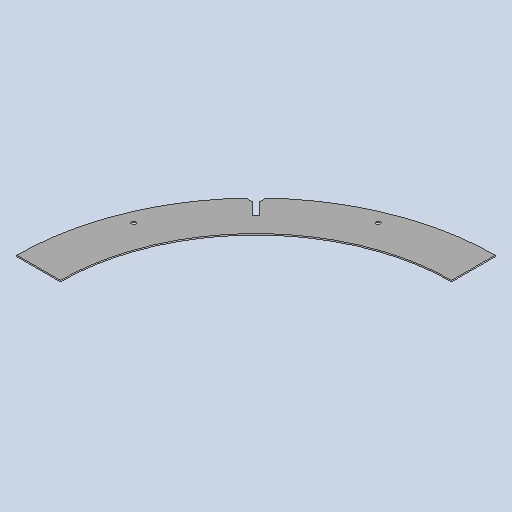
# Autodesk Inventor part: BSH 502 segment
Saved by Autodesk Inventor 2025 (Build 290162010, 162A)
## iProperties
Created: 2024-09-03
Part Number: BSH 502 segment
Material: Stainless Steel
Document SubType Name: Sheet Metal
Designer: pokla
Density: 8 g/cm^3
Flat Pattern Width: 55 cm
Flat Pattern Length: 55 cm
Flat Pattern Area: 3025 cm^2
Sheet Metal Rule: AISI304 3mm Die 32
Sheet Metal Width: 550.000 mm
Sheet Metal Length: 550.000 mm
Sheet Metal Area: 302500.000 mm^2
Appearance: Default
Mass: 1864.38 g
Surface Area: 1611.3 cm^2
Volume: 233.048 cm^3
Author: pokla
Autodesk Inventor part; units mm, degrees
ref_plane "YZ Plane" through (0, 0, 0) normal (1, 0, 0) x (0, 1, 0)
ref_plane "XZ Plane" through (0, 0, 0) normal (0, 1, 0) x (-1, 0, 0)
ref_plane "XY Plane" through (0, 0, 0) normal (0, 0, 1) x (1, 0, 0)
sketch "Sketch1" plane through (0, 0, 0) normal (0, 0, 1) x (1, 0, 0)
  arc A0 (0, 550) -> (-550, 0) centre (0, 0) ccw
  arc A1 (0, 450) -> (-450, 0) centre (0, 0) ccw
  line L0 (0, 550) -> (0, 450)
  line L1 (-450, 0) -> (-550, 0)
  point P0 (-500, 0)
  point P1 (0, 500)
  dimension "d0" = 1100
  dimension "d1" = 900
  measures "d0" diameter of A0
  measures "d1" diameter of A1
extrude "Plate1" add sketch "Sketch1" against normal blind 3
sketch "Sketch2" plane through (0, 0, 0) normal (0, 0, 1) x (1, 0, 0)
  line L0 (-550, 0) -> (-450, 0) projected
  arc A0 (0, 550) -> (-550, 0) centre (0, 0) ccw construction
  circle A1 centre (-480.4174, 198.9954) radius 5
  arc A2 (0, 450) -> (-450, 0) centre (0, 0) ccw construction
  circle A3 centre (0, 0) radius 520 construction
  line L1 (-480.4174, 198.9954) -> (0, 0) construction
  dimension "d17" = 1040
  dimension "d4" = 10
  dimension "d16" = 22.5
  constraints: 2 coincident, 2 end point, 1 centre point, 3 other
  measures "d4" diameter of A1
  measures "d16" angle of L1 L0
extrude "Cut1" cut sketch "Sketch2" against normal through all
pattern_circular "Circular Pattern1" count 2 over 45 about axis through (0, 0, 0) along (0, 0, -1) of "Cut1"
sketch "Sketch3" plane through (0, 0, 0) normal (0, 0, 1) x (1, 0, 0)
  line L0 (-388.9087, 388.9087) -> (-318.1981, 318.1981) construction
  arc A0 (0, 450) -> (-450, 0) centre (0, 0) ccw projected
  arc A1 (0, 550) -> (-550, 0) centre (0, 0) ccw projected
  line L1 (-550, 0) -> (-450, 0) projected
  line L2 (-384.6661, 393.1514) -> (-393.1514, 384.6661)
  line L3 (-384.6661, 393.1514) -> (-349.3107, 357.796)
  line L4 (-393.1514, 384.6661) -> (-357.796, 349.3107)
  line L5 (-357.796, 349.3107) -> (-349.3107, 357.796)
  point P0 (-388.9087, 388.9087)
  dimension "d11" = 45
  dimension "d12" = 12
  dimension "d13" = 50
  constraints: 10 end point, 3 point on circle, 2 line through centre, 2 parallel, 2 perpendicular, 1 midpoint
  measures "d11" angle of L1 L0
  measures "d12" distance of L2.start L2.end
  measures "d13" distance of L2.end L4.end
extrude "Extrusion1" cut sketch "Sketch3" against normal through all
chamfer "Corner Chamfer1" distance 10 angle 45 2 edges at (-384.6429, 393.1282, -1.5) (-393.1282, 384.6429, -1.5)
equation "\"d0\" = Диаметр_вн"
equation "\"d1\" = d0 - 2 * Ширина_кольца"
equation "\"d4\" = Диаметр_отв"
equation "\"d6\" = Thickness"
equation "\"d2\" = Thickness"
equation "\"BendReliefWidth\" = Thickness"
equation "\"BendReliefDepth\" = 0.5 * Thickness"
equation "\"CornerReliefSize\" = 4 * Thickness"
equation "\"MinimumRemnant\" = 2 * Thickness"
equation "\"TransitionRadius\" = BendRadius"
equation "\"JacobiRadiusSize\" = BendRadius"
equation "\"GapSize\" = Thickness"
equation "\"Диаметр_вн\" = 1100"
equation "\"Ширина_кольца\" = 100"
equation "\"Диаметр_отв\" = 10"
equation "\"Thickness\" = 3"
equation "\"BendRadius\" = 5"
body "Solid1"
